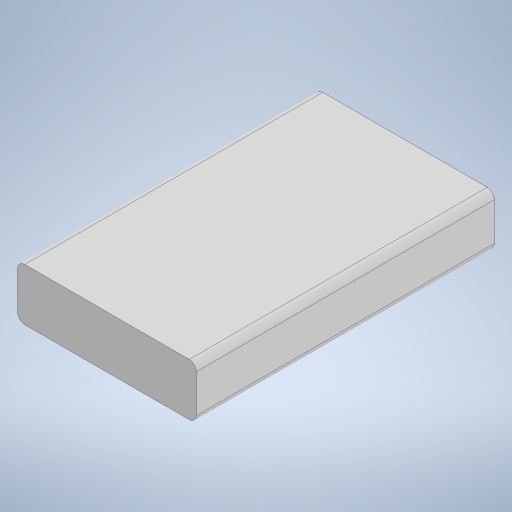
# Autodesk Inventor part: li-po 150mAh'
Saved by Autodesk Inventor 2023 (Build 270158000, 158)
## iProperties
Created: 2023-07-31
Part Number: li-po 150mAh'
Material: Ogólny
Document SubType Name: Modeling
Designer: Kamil
Density: 1 g/cm^3
Appearance: Domyślna
Author: Kamil
Autodesk Inventor part; units mm, degrees
ref_plane "YZ Plane" through (0, 0, 0) normal (1, 0, 0) x (0, 1, 0)
ref_plane "XZ Plane" through (0, 0, 0) normal (0, 1, 0) x (-1, 0, 0)
ref_plane "XY Plane" through (0, 0, 0) normal (0, 0, 1) x (1, 0, 0)
sketch "Szkic1" plane through (0, 0, 0) normal (0, 1, 0) x (-1, 0, 0)
  line L0 (0, 0) -> (15, 0)
  line L1 (15, 0) -> (15, -25)
  line L2 (15, -25) -> (0, -25)
  line L3 (0, -25) -> (0, 0)
  dimension "d0" = 15
  dimension "d1" = 25
  constraints: 8 end point, 2 parallel, 1 horizontal, 1 perpendicular
  measures "d0" distance of L1.end L2.end
  measures "d1" distance of L0.end L1.end
extrude "Wyciągnięcie proste1" add sketch "Szkic1" along normal blind 4.38
fillet "Zaokrąglenie1" radius 0.6 2 edges at (-15, 4.38, -12.5) (0, 4.38, -12.5)
fillet "Zaokrąglenie2" radius 0.6 2 edges at (-15, 0, -12.5) (0, 0, -12.5)
